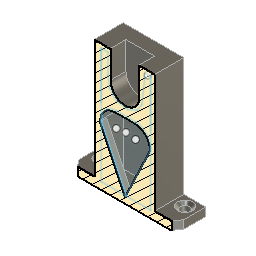
Крепление пневматического инструмента_ver4(облегченная) (Autodesk Fusion 360 design; units mm, degrees)
Autodesk Fusion 360 part; units mm, degrees
sketch "Sketch1" plane through (0, 0, 0) normal (0, 0, 1) x (1, 0, 0)
  line L0 (-5.9, 3.5) -> (-11, 3.5)
  line L1 (-11, 3.5) -> (-11, 22)
  line L2 (-11, 22) -> (0, 22)
  line L3 (5.9, 3.5) -> (11, 3.5)
  line L4 (11, 22) -> (0, 22)
  line L5 (11, 3.5) -> (11, 22)
  line L6 (-5.9, 3.5) -> (5.9, 3.5)
  line L7 (-6.1, 4.9828) -> (-6.1, 3.5)
  line L8 (-5.2, 5.8828) -> (-6.1, 4.9828)
  line L9 (-5.2, 8.2172) -> (-5.2, 5.8828)
  line L10 (-6.1, 9.1172) -> (-5.2, 8.2172)
  line L11 (-6.1, 9.1172) -> (-6.1, 10.1828)
  line L12 (-5.2, 11.0828) -> (-6.1, 10.1828)
  line L13 (-5.2, 16) -> (-5.2, 11.0828)
  line L14 (-5.2, 16) -> (-5.2, 17.2)
  line L15 (-5.2, 17.2) -> (0, 17.2)
  line L16 (5.2, 17.2) -> (0, 17.2)
  line L17 (5.2, 16) -> (5.2, 17.2)
  line L18 (5.2, 16) -> (5.2, 11.0828)
  line L19 (5.2, 11.0828) -> (6.1, 10.1828)
  line L20 (6.1, 9.1172) -> (6.1, 10.1828)
  line L21 (6.1, 9.1172) -> (5.2, 8.2172)
  line L22 (5.2, 8.2172) -> (5.2, 5.8828)
  line L23 (5.2, 5.8828) -> (6.1, 4.9828)
  line L24 (6.1, 4.9828) -> (6.1, 3.5)
  constraint perpendicular L0 L1
extrude "Extrude1" add sketch "Sketch1" along normal blind 5 contours L0 L1 L2 L3 L4 L5 L7 L8 L9 L10 L11 L12 L13 L14 L15 L16 L17 L18 L19 L20 L21 L22 L23 L24 makes body 1
extrude "Extrude2" add sketch "Sketch1" along normal blind 20 contours L0 L1 L2 L3 L4 L5 L7 L8 L9 L10 L11 L12 L13 L14 L15 L16 L17 L18 L19 L20 L21 L22 L23 L24 bodies 1
sketch "Sketch3" plane through (0, 0, 0) normal (0, 0, 1) x (1, 0, 0)
  line L0 (-5.2, 17.2) -> (-11, 17.2)
  line L1 (-6.1, 3.5) -> (-11, 3.5)
  line L2 (-11, 3.5) -> (-11, 17.2)
  line L3 (-6.1, 9.1172) -> (-6.1, 10.1828)
  line L4 (-5.2, 11.0828) -> (-6.1, 10.1828)
  line L5 (-5.2, 17.2) -> (-5.2, 11.0828)
  line L6 (-6.1, 4.9828) -> (-6.1, 3.5)
  line L7 (-5.2, 5.8828) -> (-6.1, 4.9828)
  line L8 (-5.2, 8.2172) -> (-5.2, 5.8828)
  line L9 (-6.1, 9.1172) -> (-5.2, 8.2172)
  constraint perpendicular L0 L2
revolve "Revolve1" add sketch "Sketch3" angle 360 about axis through (0, 1.75, 0) along (0, 1, 0) separate body makes body 2
sketch "Sketch4" plane through (0, 3.5, 0) normal (0, -1, 0) x (1, 0, 0)
  circle A0 centre (0, 0) radius 11
  circle A1 centre (0, 0) radius 6.1
sketch "Sketch5" plane through (0, 3.5, 0) normal (0, -1, 0) x (1, 0, 0)
  line L0 (-11, 0) -> (11, 0)
  line L1 (11, 0) -> (11, 12)
  line L2 (11, 12) -> (-11, 12)
  line L3 (-11, 12) -> (-11, 0)
  constraint horizontal L0
  constraint vertical L1
  constraint horizontal L2
  constraint vertical L3
extrude "Extrude3" cut sketch "Sketch5" against normal blind 25 bodies 2
sketch "Sketch6" plane through (0, 0, 0) normal (0, 0, -1) x (1, 0, 0)
  line L0 (-11, -3.5) -> (-11, -22)
  line L1 (-11, -22) -> (11, -22)
  line L2 (11, -22) -> (11, -3.5)
  line L3 (-6.1, -3.5) -> (-11, -3.5)
  line L4 (-11, -22) -> (11, -22)
  line L5 (11, -22) -> (11, -17.2)
  line L6 (11, -17.2) -> (-11, -17.2)
  line L7 (-11, -17.2) -> (-11, -22)
  line L8 (5.2, -8.2172) -> (6.1, -9.1172)
  line L9 (6.1, -9.1172) -> (6.1, -10.1828)
  line L10 (6.1, -10.1828) -> (5.2, -11.0828)
  line L11 (5.2, -11.0828) -> (5.2, -17.2)
  line L12 (5.2, -17.2) -> (-5.2, -17.2)
  line L13 (-5.2, -17.2) -> (-5.2, -11.0828)
  line L14 (-5.2, -11.0828) -> (-6.1, -10.1828)
  line L15 (-6.1, -10.1828) -> (-6.1, -9.1172)
  line L16 (-6.1, -9.1172) -> (-5.2, -8.2172)
  line L17 (-5.2, -8.2172) -> (-5.2, -5.8828)
  line L18 (-5.2, -5.8828) -> (-6.1, -4.9828)
  line L19 (-6.1, -4.9828) -> (-6.1, -3.5)
  line L20 (11, -3.5) -> (6.1, -3.5)
  line L21 (6.1, -3.5) -> (6.1, -4.9828)
  line L22 (6.1, -4.9828) -> (5.2, -5.8828)
  line L23 (5.2, -5.8828) -> (5.2, -8.2172)
  dimension "d40" = 4.8
  constraint horizontal L4
  constraint vertical L5
  constraint horizontal L6
  constraint vertical L7
  constraint coincident L2 L5.end
  constraint coincident L0.end L1.start
  measures "d40" distance of L1.end L5.end
extrude "Extrude4" add sketch "Sketch6" along normal blind 11 contours L0 L1 L2 L4 L5 L6 L7 L12 bodies 1
extrude "Extrude7" cut 1 faces at (-9.3667, 11.8943, 20) along direction (0, 0, -1) blind 10 on bodies 1 bodies 1 2
move_body "Move1" bodies 1 2 to x (1, 0, 0) y (0, 1, 0) z (0, 0, 1) at (0, 0, 11)
move_body "Move2" bodies 2 1 to x (1, 0, 0) y (0, 1, 0) z (0, 0, 1) at (0, -12, 0)
sketch "Sketch8" plane through (0, 5.2, 0) normal (0, -1, 0) x (1, 0, 0)
  line L0 (5.2, 21) -> (-5.2, 21)
  line L1 (-5.2, 21) -> (-5.2, 11)
  line L2 (-5.2, 11) -> (-11, 11)
  line L3 (-11, 11) -> (-11, 0)
  line L4 (-11, 0) -> (11, 0)
  line L5 (11, 0) -> (11, 11)
  line L6 (11, 11) -> (5.2, 11)
  line L7 (5.2, 11) -> (5.2, 21)
  arc A0 (-11, 11) -> (0, 0) centre (0, 11) ccw
  arc A1 (0, 0) -> (11, 11) centre (0, 11) ccw
  dimension "d41" = 11
  dimension "d42" = 11
  constraint coincident A0.end A1.start
  measures "d41" radius of A0
  measures "d42" radius of A1
extrude "Extrude8" add sketch "Sketch8" against normal blind 15 from surface at 13.7 contours L4 L5 A1 | L3 L4 A0 bodies 1 2
sketch "Sketch9" plane through (0, 0, 21) normal (0, 0, 1) x (-1, 0, 0)
  line L0 (-6.1, 2.8828) -> (-5.2, 3.7828)
  line L1 (-5.2, 3.7828) -> (-5.2, 6.1172)
  line L2 (-5.2, 6.1172) -> (-6.1, 7.0172)
  line L3 (-6.1, 7.0172) -> (-6.1, 8.5)
  line L4 (-6.1, 8.5) -> (-11, 8.5)
  line L5 (-11, 8.5) -> (-11, -10)
  line L6 (-11, -10) -> (11, -10)
  line L7 (11, -10) -> (11, 8.5)
  line L8 (11, 8.5) -> (6.1, 8.5)
  line L9 (6.1, 8.5) -> (6.1, 7.0172)
  line L10 (6.1, 7.0172) -> (5.2, 6.1172)
  line L11 (5.2, 6.1172) -> (5.2, 3.7828)
  line L12 (5.2, 3.7828) -> (6.1, 2.8828)
  line L13 (6.1, 2.8828) -> (6.1, 1.8172)
  line L14 (6.1, 1.8172) -> (5.2, 0.9172)
  line L15 (5.2, 0.9172) -> (5.2, -5.2)
  line L16 (5.2, -5.2) -> (-5.2, -5.2)
  line L17 (-5.2, -5.2) -> (-5.2, 0.9172)
  line L18 (-5.2, 0.9172) -> (-6.1, 1.8172)
  line L19 (-6.1, 1.8172) -> (-6.1, 2.8828)
extrude "Extrude11" add 1 faces at (-3.6667, 3.8333, 0) along direction (0, 0, -1) blind 25 on bodies 1 bodies 1
sketch "Sketch10" plane through (0, 0, 21) normal (0, 0, 1) x (-1, 0, 0)
  line L0 (19, -2) -> (19, -10)
  line L1 (19, -10) -> (11, -10)
  line L2 (11, -10) -> (11, 8.5)
  circle A0 centre (15, -6.5) radius 1.75
  line L3 (19, -2) -> (11, 8.5)
  line L4 (0, -1.75) -> (0, -22.5)
  line L5 (-19, -2) -> (-19, -10)
  line L6 (-11, -10) -> (-11, 8.5)
  line L7 (-19, -2) -> (-11, 8.5)
  circle A1 centre (-15, -6.5) radius 1.75
  line L8 (-19, -10) -> (-11, -10)
  dimension "d46" = 3.5
  constraint vertical L0
  constraint horizontal L1
  constraint vertical L2
  constraint symmetric L2.end L4 L6.end
  constraint symmetric L0.end L4 L5.end
  constraint symmetric L1.end L4 L6.start
  constraint symmetric A0 L4 A1
  constraint symmetric L0.start L4 L5.start
  measures "d46" diameter of A0
extrude "Extrude9" add sketch "Sketch10" along normal blind -46 and the other way blind 43 bodies 1
chamfer "Chamfer3" distance 1 angle 45 2 edges at (-13.3684, 7.1328, -22) (16.6316, 7.1328, -22) on bodies 1
shell "Shell1" thickness 2 removed faces 0 bodies 1
ref_plane "WorkPlane1" through (0, 0, -2) normal (0, -1, 0) x (1, 0, 0)
sketch "Sketch11" plane through (0, 0, 0) normal (0, -1, 0) x (-1, 0, 0)
  line L0 (0, 23) -> (9, 4)
  line L1 (9, 3.5) -> (9, 23)
  line L2 (9, 23) -> (0, 23)
  line L3 (0, 23) -> (-9, 4)
  line L4 (-9, 3.5) -> (-9, 23)
  line L5 (-9, 23) -> (0, 23)
  line L6 (9, -19) -> (9, -2)
  line L7 (3.5, -2) -> (-3.5, -2)
  line L8 (-9, -2) -> (-9, -19)
  line L9 (-9, -19) -> (-8, -19)
  line L10 (-9, -19) -> (-7, -19)
  line L11 (-7, -19) -> (-5.7584, -8.5554)
  line L12 (-5.7584, -8.5554) -> (-4, -6)
  line L13 (-4, -6) -> (-0.681, -4.5043)
  line L14 (-0.681, -4.5043) -> (3.3701, -5.2521)
  line L15 (3.3701, -5.2521) -> (6, -8)
  line L16 (6, -8) -> (6.503, -11.7423)
  line L17 (6.503, -11.7423) -> (6.503, -19)
  line L18 (6.503, -19) -> (9, -19)
  arc A0 (3.5, -2) -> (9, 3.5) centre (3.5, 3.5) ccw
  arc A1 (-9, 3.5) -> (-3.5, -2) centre (-3.5, 3.5) ccw
  line L19 (9, -19) -> (9, 4)
  line L20 (-9, -19) -> (-9, 4)
  point P0 (0, 3)
  dimension "d58" = 5.5
  constraint vertical L1
  constraint perpendicular L1 L2
  constraint perpendicular L2 L4
  constraint perpendicular L4 L5
  constraint vertical L6
  constraint perpendicular L6 L7
  constraint perpendicular L7 L8
  constraint perpendicular L8 L9
  constraint perpendicular L8 L10
  constraint vertical L17
  constraint perpendicular L6 L18
  constraint perpendicular L4 L7
  constraint coincident L1 L6.end
  constraint coincident L4 L8.start
  constraint coincident L6.end L7
  constraint tangent L7 A0
  constraint tangent L1 A0
  constraint coincident L8.start L7
  constraint tangent L7 A1
  constraint tangent L4 A1
  constraint equal A0 A1
  constraint perpendicular L18 L19
  constraint perpendicular L9 L20
  measures "d58" radius of A0
extrude "Extrude12" add sketch "Sketch11" along normal blind -9 and the other way blind -8 contours L6 L7 L8 L9 L10 L11 L12 L13 L14 L15 L16 L17 L18 A0 A1 L19 L20 bodies 1
extrude "Extrude13" add sketch "Sketch11" along normal blind -2 and the other way blind -2 contours L0 L1 L2 | L3 L4 L5 bodies 1
